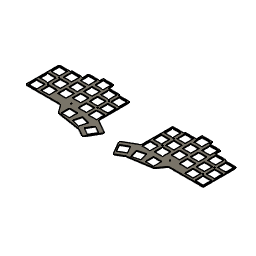
PlateV3 (Autodesk Fusion 360 design; units mm, degrees)
Autodesk Fusion 360 part; units mm, degrees
(part 1 of 4)
sketch "v1" plane through (0, 0, 0) normal (0, 1, 0) x (1, 0, 0)
  line L0 (60.175, -2.525) -> (73.175, -2.525)
  line L1 (60.175, -16.525) -> (73.175, -16.525)
  line L2 (59.675, -3.025) -> (59.675, -16.025)
  line L3 (73.675, -3.025) -> (73.675, -16.025)
  arc A0 (60.175, -2.525) -> (59.675, -3.025) centre (60.175, -3.025) ccw
  arc A1 (73.675, -3.025) -> (73.175, -2.525) centre (73.175, -3.025) ccw
  arc A2 (59.675, -16.025) -> (60.175, -16.525) centre (60.175, -16.025) ccw
  arc A3 (73.175, -16.525) -> (73.675, -16.025) centre (73.175, -16.025) ccw
  line L4 (41.125, -10.145) -> (54.125, -10.145)
  line L5 (41.125, -24.145) -> (54.125, -24.145)
  line L6 (40.625, -10.645) -> (40.625, -23.645)
  line L7 (54.625, -10.645) -> (54.625, -23.645)
  arc A4 (41.125, -10.145) -> (40.625, -10.645) centre (41.125, -10.645) ccw
  arc A5 (54.625, -10.645) -> (54.125, -10.145) centre (54.125, -10.645) ccw
  arc A6 (40.625, -23.645) -> (41.125, -24.145) centre (41.125, -23.645) ccw
  arc A7 (54.125, -24.145) -> (54.625, -23.645) centre (54.125, -23.645) ccw
  line L8 (79.225, -13.955) -> (92.225, -13.955)
  line L9 (79.225, -27.955) -> (92.225, -27.955)
  line L10 (78.725, -14.455) -> (78.725, -27.455)
  line L11 (92.725, -14.455) -> (92.725, -27.455)
  arc A8 (79.225, -13.955) -> (78.725, -14.455) centre (79.225, -14.455) ccw
  arc A9 (92.725, -14.455) -> (92.225, -13.955) centre (92.225, -14.455) ccw
  arc A10 (78.725, -27.455) -> (79.225, -27.955) centre (79.225, -27.455) ccw
  arc A11 (92.225, -27.955) -> (92.725, -27.455) centre (92.225, -27.455) ccw
  line L12 (98.275, -15.86) -> (111.275, -15.86)
  line L13 (98.275, -29.86) -> (111.275, -29.86)
  line L14 (97.775, -16.36) -> (97.775, -29.36)
  line L15 (111.775, -16.36) -> (111.775, -29.36)
  arc A12 (98.275, -15.86) -> (97.775, -16.36) centre (98.275, -16.36) ccw
  arc A13 (111.775, -16.36) -> (111.275, -15.86) centre (111.275, -16.36) ccw
  arc A14 (97.775, -29.36) -> (98.275, -29.86) centre (98.275, -29.36) ccw
  arc A15 (111.275, -29.86) -> (111.775, -29.36) centre (111.275, -29.36) ccw
  line L16 (3.025, -16.8125) -> (16.025, -16.8125)
  line L17 (3.025, -30.8125) -> (16.025, -30.8125)
  line L18 (2.525, -17.3125) -> (2.525, -30.3125)
  line L19 (16.525, -17.3125) -> (16.525, -30.3125)
  arc A16 (3.025, -16.8125) -> (2.525, -17.3125) centre (3.025, -17.3125) ccw
  arc A17 (16.525, -17.3125) -> (16.025, -16.8125) centre (16.025, -17.3125) ccw
  arc A18 (2.525, -30.3125) -> (3.025, -30.8125) centre (3.025, -30.3125) ccw
  arc A19 (16.025, -30.8125) -> (16.525, -30.3125) centre (16.025, -30.3125) ccw
  line L20 (22.075, -16.8125) -> (35.075, -16.8125)
  line L21 (22.075, -30.8125) -> (35.075, -30.8125)
  line L22 (21.575, -17.3125) -> (21.575, -30.3125)
  line L23 (35.575, -17.3125) -> (35.575, -30.3125)
  arc A20 (22.075, -16.8125) -> (21.575, -17.3125) centre (22.075, -17.3125) ccw
  arc A21 (35.575, -17.3125) -> (35.075, -16.8125) centre (35.075, -17.3125) ccw
  arc A22 (21.575, -30.3125) -> (22.075, -30.8125) centre (22.075, -30.3125) ccw
  arc A23 (35.075, -30.8125) -> (35.575, -30.3125) centre (35.075, -30.3125) ccw
  line L24 (60.175, -21.575) -> (73.175, -21.575)
  line L25 (60.175, -35.575) -> (73.175, -35.575)
  line L26 (59.675, -22.075) -> (59.675, -35.075)
  line L27 (73.675, -22.075) -> (73.675, -35.075)
  arc A24 (60.175, -21.575) -> (59.675, -22.075) centre (60.175, -22.075) ccw
  arc A25 (73.675, -22.075) -> (73.175, -21.575) centre (73.175, -22.075) ccw
  arc A26 (59.675, -35.075) -> (60.175, -35.575) centre (60.175, -35.075) ccw
  arc A27 (73.175, -35.575) -> (73.675, -35.075) centre (73.175, -35.075) ccw
  line L28 (41.125, -29.195) -> (54.125, -29.195)
  line L29 (41.125, -43.195) -> (54.125, -43.195)
  line L30 (40.625, -29.695) -> (40.625, -42.695)
  line L31 (54.625, -29.695) -> (54.625, -42.695)
  arc A28 (41.125, -29.195) -> (40.625, -29.695) centre (41.125, -29.695) ccw
  arc A29 (54.625, -29.695) -> (54.125, -29.195) centre (54.125, -29.695) ccw
  arc A30 (40.625, -42.695) -> (41.125, -43.195) centre (41.125, -42.695) ccw
  arc A31 (54.125, -43.195) -> (54.625, -42.695) centre (54.125, -42.695) ccw
  line L32 (79.225, -33.005) -> (92.225, -33.005)
  line L33 (79.225, -47.005) -> (92.225, -47.005)
  line L34 (78.725, -33.505) -> (78.725, -46.505)
  line L35 (92.725, -33.505) -> (92.725, -46.505)
  arc A32 (79.225, -33.005) -> (78.725, -33.505) centre (79.225, -33.505) ccw
  arc A33 (92.725, -33.505) -> (92.225, -33.005) centre (92.225, -33.505) ccw
  arc A34 (78.725, -46.505) -> (79.225, -47.005) centre (79.225, -46.505) ccw
  arc A35 (92.225, -47.005) -> (92.725, -46.505) centre (92.225, -46.505) ccw
  line L36 (98.275, -34.91) -> (111.275, -34.91)
  line L37 (98.275, -48.91) -> (111.275, -48.91)
  line L38 (97.775, -35.41) -> (97.775, -48.41)
  line L39 (111.775, -35.41) -> (111.775, -48.41)
  arc A36 (98.275, -34.91) -> (97.775, -35.41) centre (98.275, -35.41) ccw
  arc A37 (111.775, -35.41) -> (111.275, -34.91) centre (111.275, -35.41) ccw
  arc A38 (97.775, -48.41) -> (98.275, -48.91) centre (98.275, -48.41) ccw
  arc A39 (111.275, -48.91) -> (111.775, -48.41) centre (111.275, -48.41) ccw
  line L40 (3.025, -35.8625) -> (16.025, -35.8625)
  line L41 (3.025, -49.8625) -> (16.025, -49.8625)
  line L42 (2.525, -36.3625) -> (2.525, -49.3625)
  line L43 (16.525, -36.3625) -> (16.525, -49.3625)
  arc A40 (3.025, -35.8625) -> (2.525, -36.3625) centre (3.025, -36.3625) ccw
  arc A41 (16.525, -36.3625) -> (16.025, -35.8625) centre (16.025, -36.3625) ccw
  arc A42 (2.525, -49.3625) -> (3.025, -49.8625) centre (3.025, -49.3625) ccw
  arc A43 (16.025, -49.8625) -> (16.525, -49.3625) centre (16.025, -49.3625) ccw
  line L44 (22.075, -35.8625) -> (35.075, -35.8625)
  line L45 (22.075, -49.8625) -> (35.075, -49.8625)
  line L46 (21.575, -36.3625) -> (21.575, -49.3625)
  line L47 (35.575, -36.3625) -> (35.575, -49.3625)
  arc A44 (22.075, -35.8625) -> (21.575, -36.3625) centre (22.075, -36.3625) ccw
  arc A45 (35.575, -36.3625) -> (35.075, -35.8625) centre (35.075, -36.3625) ccw
  arc A46 (21.575, -49.3625) -> (22.075, -49.8625) centre (22.075, -49.3625) ccw
  arc A47 (35.075, -49.8625) -> (35.575, -49.3625) centre (35.075, -49.3625) ccw
  line L48 (60.175, -40.625) -> (73.175, -40.625)
  line L49 (60.175, -54.625) -> (73.175, -54.625)
  line L50 (59.675, -41.125) -> (59.675, -54.125)
  line L51 (73.675, -41.125) -> (73.675, -54.125)
  arc A48 (60.175, -40.625) -> (59.675, -41.125) centre (60.175, -41.125) ccw
  arc A49 (73.675, -41.125) -> (73.175, -40.625) centre (73.175, -41.125) ccw
  arc A50 (59.675, -54.125) -> (60.175, -54.625) centre (60.175, -54.125) ccw
  arc A51 (73.175, -54.625) -> (73.675, -54.125) centre (73.175, -54.125) ccw
  line L52 (41.125, -48.245) -> (54.125, -48.245)
  line L53 (41.125, -62.245) -> (54.125, -62.245)
  line L54 (40.625, -48.745) -> (40.625, -61.745)
  line L55 (54.625, -48.745) -> (54.625, -61.745)
  arc A52 (41.125, -48.245) -> (40.625, -48.745) centre (41.125, -48.745) ccw
  arc A53 (54.625, -48.745) -> (54.125, -48.245) centre (54.125, -48.745) ccw
  arc A54 (40.625, -61.745) -> (41.125, -62.245) centre (41.125, -61.745) ccw
  arc A55 (54.125, -62.245) -> (54.625, -61.745) centre (54.125, -61.745) ccw
  line L56 (79.225, -52.055) -> (92.225, -52.055)
  line L57 (79.225, -66.055) -> (92.225, -66.055)
  line L58 (78.725, -52.555) -> (78.725, -65.555)
  line L59 (92.725, -52.555) -> (92.725, -65.555)
  arc A56 (79.225, -52.055) -> (78.725, -52.555) centre (79.225, -52.555) ccw
  arc A57 (92.725, -52.555) -> (92.225, -52.055) centre (92.225, -52.555) ccw
  arc A58 (78.725, -65.555) -> (79.225, -66.055) centre (79.225, -65.555) ccw
  arc A59 (92.225, -66.055) -> (92.725, -65.555) centre (92.225, -65.555) ccw
  line L60 (98.275, -53.96) -> (111.275, -53.96)
  line L61 (98.275, -67.96) -> (111.275, -67.96)
  line L62 (97.775, -54.46) -> (97.775, -67.46)
  line L63 (111.775, -54.46) -> (111.775, -67.46)
  arc A60 (98.275, -53.96) -> (97.775, -54.46) centre (98.275, -54.46) ccw
  arc A61 (111.775, -54.46) -> (111.275, -53.96) centre (111.275, -54.46) ccw
  arc A62 (97.775, -67.46) -> (98.275, -67.96) centre (98.275, -67.46) ccw
  arc A63 (111.275, -67.96) -> (111.775, -67.46) centre (111.275, -67.46) ccw
  line L64 (3.025, -54.9125) -> (16.025, -54.9125)
  line L65 (3.025, -68.9125) -> (16.025, -68.9125)
  line L66 (2.525, -55.4125) -> (2.525, -68.4125)
  line L67 (16.525, -55.4125) -> (16.525, -68.4125)
  arc A64 (3.025, -54.9125) -> (2.525, -55.4125) centre (3.025, -55.4125) ccw
  arc A65 (16.525, -55.4125) -> (16.025, -54.9125) centre (16.025, -55.4125) ccw
  arc A66 (2.525, -68.4125) -> (3.025, -68.9125) centre (3.025, -68.4125) ccw
  arc A67 (16.025, -68.9125) -> (16.525, -68.4125) centre (16.025, -68.4125) ccw
  line L68 (22.075, -54.9125) -> (35.075, -54.9125)
  line L69 (22.075, -68.9125) -> (35.075, -68.9125)
  line L70 (21.575, -55.4125) -> (21.575, -68.4125)
  line L71 (35.575, -55.4125) -> (35.575, -68.4125)
  arc A68 (22.075, -54.9125) -> (21.575, -55.4125) centre (22.075, -55.4125) ccw
  arc A69 (35.575, -55.4125) -> (35.075, -54.9125) centre (35.075, -55.4125) ccw
  arc A70 (21.575, -68.4125) -> (22.075, -68.9125) centre (22.075, -68.4125) ccw
  arc A71 (35.075, -68.9125) -> (35.575, -68.4125) centre (35.075, -68.4125) ccw
  line L72 (69.7, -73.9625) -> (82.7, -73.9625)
  line L73 (69.7, -87.9625) -> (82.7, -87.9625)
  line L74 (69.2, -74.4625) -> (69.2, -87.4625)
  line L75 (83.2, -74.4625) -> (83.2, -87.4625)
  arc A72 (69.7, -73.9625) -> (69.2, -74.4625) centre (69.7, -74.4625) ccw
  arc A73 (83.2, -74.4625) -> (82.7, -73.9625) centre (82.7, -74.4625) ccw
  arc A74 (69.2, -87.4625) -> (69.7, -87.9625) centre (69.7, -87.4625) ccw
  arc A75 (82.7, -87.9625) -> (83.2, -87.4625) centre (82.7, -87.4625) ccw
  line L76 (94.5706, -75.2238) -> (107.1276, -78.5884)
  line L77 (90.9471, -88.7468) -> (103.5041, -92.1114)
  line L78 (93.9582, -75.5774) -> (90.5936, -88.1344)
  line L79 (107.4812, -79.2008) -> (104.1165, -91.7579)
  arc A76 (94.5706, -75.2238) -> (93.9582, -75.5774) centre (94.4412, -75.7068) ccw
  arc A77 (107.4812, -79.2008) -> (107.1276, -78.5884) centre (106.9982, -79.0714) ccw
  arc A78 (90.5936, -88.1344) -> (90.9471, -88.7468) centre (91.0765, -88.2638) ccw
  arc A79 (103.5041, -92.1114) -> (104.1165, -91.7579) centre (103.6336, -91.6284) ccw
  line L80 (132.3373, -85.6651) -> (125.8373, -96.9234)
  line L81 (120.213, -78.6651) -> (113.713, -89.9234)
  line L82 (132.1543, -84.9821) -> (120.896, -78.4821)
  line L83 (125.1543, -97.1064) -> (113.896, -90.6064)
  arc A80 (132.3373, -85.6651) -> (132.1543, -84.9821) centre (131.9043, -85.4151) ccw
  arc A81 (125.1543, -97.1064) -> (125.8373, -96.9234) centre (125.4043, -96.6734) ccw
  arc A82 (120.896, -78.4821) -> (120.213, -78.6651) centre (120.646, -78.9151) ccw
  arc A83 (113.713, -89.9234) -> (113.896, -90.6064) centre (114.146, -90.1734) ccw
  line L84 (1.025, -14.8125) -> (16.025, -14.8125)
  line L85 (22.075, -14.8125) -> (38.125, -14.8125)
  line L86 (41.125, -8.145) -> (57.175, -8.145)
  line L87 (58.175, -0.525) -> (73.175, -0.525)
  line L88 (76.175, -11.955) -> (92.225, -11.955)
  line L89 (95.225, -13.86) -> (113.275, -13.86)
  line L90 (113.775, -35.41) -> (113.775, -48.41)
  line L91 (113.775, -14.36) -> (113.775, -29.36)
  line L92 (113.775, -54.46) -> (113.775, -70.3293)
  line L93 (134.8864, -84.25) -> (115.275, -72.9274)
  line L94 (135.0694, -84.933) -> (126.4078, -99.9353)
  line L95 (88.3927, -90.1329) -> (102.9865, -94.0433)
  line L96 (70.2949, -89.9625) -> (87.0986, -89.9625)
  line L97 (22.075, -70.9125) -> (35.1033, -70.9125)
  line L98 (1.025, -70.9125) -> (16.025, -70.9125)
  line L99 (0.525, -55.4125) -> (0.525, -70.4125)
  line L100 (0.525, -36.3625) -> (0.525, -49.3625)
  line L101 (0.525, -15.3125) -> (0.525, -30.3125)
  line L102 (0.525, -30.3125) -> (0.525, -36.3625)
  line L103 (0.525, -49.3625) -> (0.525, -55.4125)
  line L104 (16.025, -70.9125) -> (22.075, -70.9125)
  line L105 (113.775, -54.46) -> (113.775, -48.41)
  line L106 (113.775, -35.41) -> (113.775, -29.36)
  line L107 (16.025, -14.8125) -> (22.075, -14.8125)
  line L108 (70.5671, -89.9625) -> (68.5671, -89.9625)
  line L109 (35.1033, -70.9125) -> (37.1033, -70.9125)
  line L110 (37.1033, -70.9125) -> (54.6027, -70.8754)
  line L111 (58.9382, -73.3662) -> (67.7, -88.468)
  line L112 (102.9865, -94.0433) -> (125.8454, -100.1683)
  line L113 (126.216, -100.2676) -> (127.5694, -97.9234)
  arc A84 (88.3927, -90.1329) -> (87.0986, -89.9625) centre (87.0986, -94.9625) ccw
  arc A85 (135.0694, -84.933) -> (134.8864, -84.25) centre (134.6364, -84.683) ccw
  arc A86 (113.775, -70.3293) -> (115.275, -72.9274) centre (116.775, -70.3293) ccw
  arc A87 (113.775, -14.36) -> (113.275, -13.86) centre (113.275, -14.36) ccw
  arc A88 (58.9382, -73.3662) -> (54.6027, -70.8754) centre (54.6133, -75.8753) ccw
  arc A89 (67.7, -88.468) -> (70.2949, -89.9625) centre (70.2949, -86.9625) ccw
  arc A90 (0.525, -70.4125) -> (1.025, -70.9125) centre (1.025, -70.4125) ccw
  arc A91 (1.025, -14.8125) -> (0.525, -15.3125) centre (1.025, -15.3125) ccw
  arc A92 (125.8454, -100.1683) -> (126.4078, -99.9353) centre (125.9748, -99.6853) ccw
  line L114 (38.625, -14.3125) -> (38.625, -8.645)
  line L115 (41.125, -8.145) -> (39.125, -8.145)
  line L116 (57.675, -7.645) -> (57.675, -1.025)
  line L117 (57.675, -0.525) -> (60.175, -0.525)
  line L118 (75.675, -11.455) -> (75.675, -1.025)
  line L119 (75.175, -0.525) -> (73.175, -0.525)
  line L120 (94.725, -13.36) -> (94.725, -12.455)
  line L121 (94.225, -11.955) -> (92.225, -11.955)
  arc A93 (38.125, -14.8125) -> (38.625, -14.3125) centre (38.125, -14.3125) ccw
  arc A94 (39.125, -8.145) -> (38.625, -8.645) centre (39.125, -8.645) ccw
  arc A95 (57.175, -8.145) -> (57.675, -7.645) centre (57.175, -7.645) ccw
  arc A96 (58.175, -0.525) -> (57.675, -1.025) centre (58.175, -1.025) ccw
  arc A97 (75.675, -1.025) -> (75.175, -0.525) centre (75.175, -1.025) ccw
  arc A98 (94.725, -12.455) -> (94.225, -11.955) centre (94.225, -12.455) ccw
  arc A99 (75.675, -11.455) -> (76.175, -11.955) centre (76.175, -11.455) ccw
  arc A100 (94.725, -13.36) -> (95.225, -13.86) centre (95.225, -13.36) ccw
  arc A101 (169.0598, -78.6651) -> (168.3767, -78.4821) centre (168.6267, -78.9151) ccw
  arc A102 (157.1184, -84.9821) -> (156.9354, -85.6651) centre (157.3684, -85.4151) ccw
  line L122 (181.7916, -79.2008) -> (185.1562, -91.7579)
  line L123 (154.3864, -84.25) -> (173.9977, -72.9274)
  line L124 (156.9354, -85.6651) -> (163.4354, -96.9234)
  arc A103 (162.8649, -99.9353) -> (163.4273, -100.1683) centre (163.2979, -99.6853) ccw
  arc A104 (190.9977, -67.96) -> (191.4977, -67.46) centre (190.9977, -67.46) ccw
  line L125 (230.3346, -73.3662) -> (221.5727, -88.468)
  line L126 (163.0567, -100.2676) -> (161.7033, -97.9234)
  line L127 (154.2033, -84.933) -> (162.8649, -99.9353)
  line L128 (229.0977, -2.525) -> (216.0977, -2.525)
  arc A105 (177.9977, -53.96) -> (177.4977, -54.46) centre (177.9977, -54.46) ccw
  line L129 (157.1184, -84.9821) -> (168.3767, -78.4821)
  line L130 (229.0977, -16.525) -> (216.0977, -16.525)
  line L131 (190.9977, -67.96) -> (177.9977, -67.96)
  line L132 (229.0977, -54.625) -> (216.0977, -54.625)
  line L133 (196.5477, -33.505) -> (196.5477, -46.505)
  line L134 (190.9977, -48.91) -> (177.9977, -48.91)
  line L135 (229.0977, -21.575) -> (216.0977, -21.575)
  line L136 (229.0977, -40.625) -> (216.0977, -40.625)
  line L137 (253.6977, -36.3625) -> (253.6977, -49.3625)
  line L138 (229.5977, -41.125) -> (229.5977, -54.125)
  line L139 (267.6977, -36.3625) -> (267.6977, -49.3625)
  line L140 (215.5977, -41.125) -> (215.5977, -54.125)
  line L141 (210.5477, -33.505) -> (210.5477, -46.505)
  line L142 (288.7477, -36.3625) -> (288.7477, -49.3625)
  line L143 (177.4977, -35.41) -> (177.4977, -48.41)
  line L144 (175.4977, -35.41) -> (175.4977, -48.41)
  line L145 (286.7477, -36.3625) -> (286.7477, -49.3625)
  line L146 (194.7021, -75.2238) -> (182.1451, -78.5884)
  line L147 (272.7477, -36.3625) -> (272.7477, -49.3625)
  line L148 (191.4977, -35.41) -> (191.4977, -48.41)
  line L149 (164.1184, -97.1064) -> (175.3767, -90.6064)
  line L150 (190.9977, -53.96) -> (177.9977, -53.96)
  arc A106 (177.4977, -48.41) -> (177.9977, -48.91) centre (177.9977, -48.41) ccw
  line L151 (248.1477, -29.195) -> (235.1477, -29.195)
  arc A107 (267.1977, -68.9125) -> (267.6977, -68.4125) centre (267.1977, -68.4125) ccw
  line L152 (288.7477, -49.3625) -> (288.7477, -55.4125)
  arc A108 (272.7477, -68.4125) -> (273.2477, -68.9125) centre (273.2477, -68.4125) ccw
  arc A109 (196.5477, -27.455) -> (197.0477, -27.955) centre (197.0477, -27.455) ccw
  line L153 (288.7477, -15.3125) -> (288.7477, -30.3125)
  line L154 (210.0477, -33.005) -> (197.0477, -33.005)
  line L155 (286.2477, -16.8125) -> (273.2477, -16.8125)
  arc A110 (248.6477, -10.645) -> (248.1477, -10.145) centre (248.1477, -10.645) ccw
  arc A111 (213.0977, -11.955) -> (213.5977, -11.455) centre (213.0977, -11.455) ccw
  arc A112 (215.5977, -35.075) -> (216.0977, -35.575) centre (216.0977, -35.075) ccw
  arc A113 (210.0477, -47.005) -> (210.5477, -46.505) centre (210.0477, -46.505) ccw
  line L156 (288.2477, -70.9125) -> (273.2477, -70.9125)
  line L157 (272.7477, -17.3125) -> (272.7477, -30.3125)
  arc A114 (267.1977, -30.8125) -> (267.6977, -30.3125) centre (267.1977, -30.3125) ccw
  line L158 (286.7477, -17.3125) -> (286.7477, -30.3125)
  arc A115 (197.0477, -52.055) -> (196.5477, -52.555) centre (197.0477, -52.555) ccw
  line L159 (213.0977, -11.955) -> (197.0477, -11.955)
  arc A116 (267.6977, -17.3125) -> (267.1977, -16.8125) centre (267.1977, -17.3125) ccw
  arc A117 (272.7477, -30.3125) -> (273.2477, -30.8125) centre (273.2477, -30.3125) ccw
  line L160 (229.5977, -3.025) -> (229.5977, -16.025)
  arc A118 (273.2477, -16.8125) -> (272.7477, -17.3125) centre (273.2477, -17.3125) ccw
  arc A119 (273.2477, -54.9125) -> (272.7477, -55.4125) centre (273.2477, -55.4125) ccw
  line L161 (215.5977, -3.025) -> (215.5977, -16.025)
  line L162 (210.0477, -27.955) -> (197.0477, -27.955)
  arc A120 (216.0977, -40.625) -> (215.5977, -41.125) centre (216.0977, -41.125) ccw
  arc A121 (235.1477, -10.145) -> (234.6477, -10.645) centre (235.1477, -10.645) ccw
  arc A122 (210.0477, -27.955) -> (210.5477, -27.455) centre (210.0477, -27.455) ccw
  line L163 (288.7477, -30.3125) -> (288.7477, -36.3625)
  arc A123 (286.2477, -30.8125) -> (286.7477, -30.3125) centre (286.2477, -30.3125) ccw
  line L164 (273.2477, -14.8125) -> (267.1977, -14.8125)
  arc A124 (254.1977, -16.8125) -> (253.6977, -17.3125) centre (254.1977, -17.3125) ccw
  line L165 (229.5977, -22.075) -> (229.5977, -35.075)
  arc A125 (253.6977, -30.3125) -> (254.1977, -30.8125) centre (254.1977, -30.3125) ccw
  arc A126 (286.7477, -17.3125) -> (286.2477, -16.8125) centre (286.2477, -17.3125) ccw
  arc A127 (254.1977, -35.8625) -> (253.6977, -36.3625) centre (254.1977, -36.3625) ccw
  line L166 (288.2477, -14.8125) -> (273.2477, -14.8125)
  arc A128 (248.6477, -29.695) -> (248.1477, -29.195) centre (248.1477, -29.695) ccw
  arc A129 (250.6477, -14.3125) -> (251.1477, -14.8125) centre (251.1477, -14.3125) ccw
  line L167 (234.6477, -10.645) -> (234.6477, -23.645)
  arc A130 (231.5977, -7.645) -> (232.0977, -8.145) centre (232.0977, -7.645) ccw
  arc A131 (288.7477, -15.3125) -> (288.2477, -14.8125) centre (288.2477, -15.3125) ccw
  line L168 (267.6977, -17.3125) -> (267.6977, -30.3125)
  arc A132 (210.5477, -33.505) -> (210.0477, -33.005) centre (210.0477, -33.505) ccw
  line L169 (248.1477, -8.145) -> (232.0977, -8.145)
  line L170 (286.2477, -35.8625) -> (273.2477, -35.8625)
  arc A133 (229.5977, -22.075) -> (229.0977, -21.575) centre (229.0977, -22.075) ccw
  line L171 (253.6977, -17.3125) -> (253.6977, -30.3125)
  line L172 (248.6477, -10.645) -> (248.6477, -23.645)
  line L173 (248.1477, -8.145) -> (250.1477, -8.145)
  arc A134 (248.1477, -43.195) -> (248.6477, -42.695) centre (248.1477, -42.695) ccw
  line L174 (231.5977, -7.645) -> (231.5977, -1.025)
  arc A135 (248.1477, -24.145) -> (248.6477, -23.645) centre (248.1477, -23.645) ccw
  line L175 (231.5977, -0.525) -> (229.0977, -0.525)
  arc A136 (234.6477, -42.695) -> (235.1477, -43.195) centre (235.1477, -42.695) ccw
  arc A137 (235.1477, -29.195) -> (234.6477, -29.695) centre (235.1477, -29.695) ccw
  line L176 (234.6477, -29.695) -> (234.6477, -42.695)
  arc A138 (229.5977, -41.125) -> (229.0977, -40.625) centre (229.0977, -41.125) ccw
  line L177 (250.6477, -14.3125) -> (250.6477, -8.645)
  arc A139 (229.0977, -16.525) -> (229.5977, -16.025) centre (229.0977, -16.025) ccw
  line L178 (248.1477, -10.145) -> (235.1477, -10.145)
  arc A140 (229.0977, -35.575) -> (229.5977, -35.075) centre (229.0977, -35.075) ccw
  arc A141 (231.5977, -1.025) -> (231.0977, -0.525) centre (231.0977, -1.025) ccw
  line L179 (248.6477, -29.695) -> (248.6477, -42.695)
  arc A142 (173.9977, -72.9274) -> (175.4977, -70.3293) centre (172.4977, -70.3293) ccw
  line L180 (175.4977, -54.46) -> (175.4977, -48.41)
  arc A143 (185.1562, -91.7579) -> (185.7686, -92.1114) centre (185.6392, -91.6284) ccw
  arc A144 (191.4977, -54.46) -> (190.9977, -53.96) centre (190.9977, -54.46) ccw
  line L181 (169.0598, -78.6651) -> (175.5598, -89.9234)
  arc A145 (154.3864, -84.25) -> (154.2033, -84.933) centre (154.6364, -84.683) ccw
  line L182 (177.4977, -54.46) -> (177.4977, -67.46)
  line L183 (190.9977, -29.86) -> (177.9977, -29.86)
  line L184 (267.1977, -68.9125) -> (254.1977, -68.9125)
  line L185 (267.1977, -54.9125) -> (254.1977, -54.9125)
  line L186 (267.1977, -30.8125) -> (254.1977, -30.8125)
  line L187 (267.1977, -49.8625) -> (254.1977, -49.8625)
  line L188 (210.0477, -47.005) -> (197.0477, -47.005)
  line L189 (195.0477, -11.955) -> (197.0477, -11.955)
  line L190 (248.6477, -48.745) -> (248.6477, -61.745)
  arc A146 (196.5477, -65.555) -> (197.0477, -66.055) centre (197.0477, -65.555) ccw
  line L191 (218.7056, -89.9625) -> (220.7056, -89.9625)
  arc A147 (195.3145, -75.5774) -> (194.7021, -75.2238) centre (194.8316, -75.7068) ccw
  line L192 (267.1977, -16.8125) -> (254.1977, -16.8125)
  arc A148 (215.5977, -54.125) -> (216.0977, -54.625) centre (216.0977, -54.125) ccw
  arc A149 (253.6977, -49.3625) -> (254.1977, -49.8625) centre (254.1977, -49.3625) ccw
  line L193 (215.5977, -22.075) -> (215.5977, -35.075)
  line L194 (200.88, -90.1329) -> (186.2862, -94.0433)
  arc A150 (195.0477, -11.955) -> (194.5477, -12.455) centre (195.0477, -12.455) ccw
  line L195 (196.5477, -14.455) -> (196.5477, -27.455)
  arc A151 (177.9977, -15.86) -> (177.4977, -16.36) centre (177.9977, -16.36) ccw
  line L196 (198.3256, -88.7468) -> (185.7686, -92.1114)
  line L197 (194.0477, -13.86) -> (175.9977, -13.86)
  arc A152 (229.0977, -54.625) -> (229.5977, -54.125) centre (229.0977, -54.125) ccw
  line L198 (267.1977, -70.9125) -> (254.1694, -70.9125)
  line L199 (195.3145, -75.5774) -> (198.6792, -88.1344)
  line L200 (286.2477, -68.9125) -> (273.2477, -68.9125)
  line L201 (219.5727, -73.9625) -> (206.5727, -73.9625)
  line L202 (248.1477, -62.245) -> (235.1477, -62.245)
  arc A153 (197.0477, -33.005) -> (196.5477, -33.505) centre (197.0477, -33.505) ccw
  arc A154 (267.1977, -49.8625) -> (267.6977, -49.3625) centre (267.1977, -49.3625) ccw
  arc A155 (234.6477, -61.745) -> (235.1477, -62.245) centre (235.1477, -61.745) ccw
  arc A156 (198.3256, -88.7468) -> (198.6792, -88.1344) centre (198.1962, -88.2638) ccw
  arc A157 (191.4977, -16.36) -> (190.9977, -15.86) centre (190.9977, -16.36) ccw
  arc A158 (286.2477, -68.9125) -> (286.7477, -68.4125) centre (286.2477, -68.4125) ccw
  line L203 (175.4977, -14.36) -> (175.4977, -29.36)
  line L204 (194.5477, -13.36) -> (194.5477, -12.455)
  line L205 (267.1977, -14.8125) -> (251.1477, -14.8125)
  line L206 (234.6477, -48.745) -> (234.6477, -61.745)
  arc A159 (194.0477, -13.86) -> (194.5477, -13.36) centre (194.0477, -13.36) ccw
  line L207 (267.1977, -35.8625) -> (254.1977, -35.8625)
  line L208 (286.2477, -30.8125) -> (273.2477, -30.8125)
  arc A160 (177.9977, -34.91) -> (177.4977, -35.41) centre (177.9977, -35.41) ccw
  arc A161 (248.1477, -62.245) -> (248.6477, -61.745) centre (248.1477, -61.745) ccw
  line L209 (210.5477, -52.555) -> (210.5477, -65.555)
  arc A162 (248.6477, -48.745) -> (248.1477, -48.245) centre (248.1477, -48.745) ccw
  arc A163 (196.5477, -46.505) -> (197.0477, -47.005) centre (197.0477, -46.505) ccw
  line L210 (219.5727, -87.9625) -> (206.5727, -87.9625)
  arc A164 (190.9977, -29.86) -> (191.4977, -29.36) centre (190.9977, -29.36) ccw
  arc A165 (220.0727, -74.4625) -> (219.5727, -73.9625) centre (219.5727, -74.4625) ccw
  line L211 (175.4977, -35.41) -> (175.4977, -29.36)
  arc A166 (254.1977, -54.9125) -> (253.6977, -55.4125) centre (254.1977, -55.4125) ccw
  line L212 (253.6977, -55.4125) -> (253.6977, -68.4125)
  arc A167 (216.0977, -21.575) -> (215.5977, -22.075) centre (216.0977, -22.075) ccw
  line L213 (288.7477, -55.4125) -> (288.7477, -70.4125)
  line L214 (252.1694, -70.9125) -> (234.67, -70.8754)
  arc A168 (218.9778, -89.9625) -> (221.5727, -88.468) centre (218.9778, -86.9625) ccw
  line L215 (248.1477, -48.245) -> (235.1477, -48.245)
  line L216 (196.5477, -52.555) -> (196.5477, -65.555)
  line L217 (272.7477, -55.4125) -> (272.7477, -68.4125)
  arc A169 (253.6977, -68.4125) -> (254.1977, -68.9125) centre (254.1977, -68.4125) ccw
  arc A170 (234.67, -70.8754) -> (230.3346, -73.3662) centre (234.6594, -75.8753) ccw
  line L218 (286.7477, -55.4125) -> (286.7477, -68.4125)
  arc A171 (210.0477, -66.055) -> (210.5477, -65.555) centre (210.0477, -65.555) ccw
  arc A172 (216.0977, -2.525) -> (215.5977, -3.025) centre (216.0977, -3.025) ccw
  arc A173 (191.4977, -35.41) -> (190.9977, -34.91) centre (190.9977, -35.41) ccw
  arc A174 (286.7477, -55.4125) -> (286.2477, -54.9125) centre (286.2477, -55.4125) ccw
  line L219 (190.9977, -34.91) -> (177.9977, -34.91)
  line L220 (254.1694, -70.9125) -> (252.1694, -70.9125)
  line L221 (286.2477, -49.8625) -> (273.2477, -49.8625)
  arc A175 (175.9977, -13.86) -> (175.4977, -14.36) centre (175.9977, -14.36) ccw
  arc A176 (177.4977, -29.36) -> (177.9977, -29.86) centre (177.9977, -29.36) ccw
  line L222 (218.9778, -89.9625) -> (202.1741, -89.9625)
  line L223 (220.0727, -74.4625) -> (220.0727, -87.4625)
  line L224 (210.0477, -13.955) -> (197.0477, -13.955)
  arc A177 (219.5727, -87.9625) -> (220.0727, -87.4625) centre (219.5727, -87.4625) ccw
  arc A178 (286.7477, -36.3625) -> (286.2477, -35.8625) centre (286.2477, -36.3625) ccw
  line L225 (214.0977, -0.525) -> (216.0977, -0.525)
  line L226 (248.1477, -43.195) -> (235.1477, -43.195)
  arc A179 (214.0977, -0.525) -> (213.5977, -1.025) centre (214.0977, -1.025) ccw
  arc A180 (229.5977, -3.025) -> (229.0977, -2.525) centre (229.0977, -3.025) ccw
  arc A181 (288.2477, -70.9125) -> (288.7477, -70.4125) centre (288.2477, -70.4125) ccw
  line L227 (248.1477, -24.145) -> (235.1477, -24.145)
  line L228 (213.5977, -11.455) -> (213.5977, -1.025)
  line L229 (190.9977, -15.86) -> (177.9977, -15.86)
  arc A182 (210.5477, -52.555) -> (210.0477, -52.055) centre (210.0477, -52.555) ccw
  line L230 (206.0727, -74.4625) -> (206.0727, -87.4625)
  arc A183 (235.1477, -48.245) -> (234.6477, -48.745) centre (235.1477, -48.745) ccw
  line L231 (210.0477, -52.055) -> (197.0477, -52.055)
  arc A184 (215.5977, -16.025) -> (216.0977, -16.525) centre (216.0977, -16.025) ccw
  line L232 (177.4977, -16.36) -> (177.4977, -29.36)
  arc A185 (197.0477, -13.955) -> (196.5477, -14.455) centre (197.0477, -14.455) ccw
  arc A186 (206.5727, -73.9625) -> (206.0727, -74.4625) centre (206.5727, -74.4625) ccw
  arc A187 (267.6977, -55.4125) -> (267.1977, -54.9125) centre (267.1977, -55.4125) ccw
  line L233 (191.4977, -16.36) -> (191.4977, -29.36)
  arc A188 (273.2477, -35.8625) -> (272.7477, -36.3625) centre (273.2477, -36.3625) ccw
  arc A189 (286.2477, -49.8625) -> (286.7477, -49.3625) centre (286.2477, -49.3625) ccw
  line L234 (273.2477, -70.9125) -> (267.1977, -70.9125)
  arc A190 (206.0727, -87.4625) -> (206.5727, -87.9625) centre (206.5727, -87.4625) ccw
  arc A191 (272.7477, -49.3625) -> (273.2477, -49.8625) centre (273.2477, -49.3625) ccw
  arc A192 (267.6977, -36.3625) -> (267.1977, -35.8625) centre (267.1977, -36.3625) ccw
  arc A193 (202.1741, -89.9625) -> (200.88, -90.1329) centre (202.1741, -94.9625) ccw
  line L235 (286.2477, -54.9125) -> (273.2477, -54.9125)
  line L236 (267.6977, -55.4125) -> (267.6977, -68.4125)
  line L237 (210.0477, -66.055) -> (197.0477, -66.055)
  arc A194 (250.6477, -8.645) -> (250.1477, -8.145) centre (250.1477, -8.645) ccw
  arc A195 (234.6477, -23.645) -> (235.1477, -24.145) centre (235.1477, -23.645) ccw
  arc A196 (210.5477, -14.455) -> (210.0477, -13.955) centre (210.0477, -14.455) ccw
  line L238 (210.5477, -14.455) -> (210.5477, -27.455)
  arc A197 (177.4977, -67.46) -> (177.9977, -67.96) centre (177.9977, -67.46) ccw
  line L239 (229.0977, -35.575) -> (216.0977, -35.575)
  arc A198 (163.4354, -96.9234) -> (164.1184, -97.1064) centre (163.8684, -96.6734) ccw
  arc A199 (190.9977, -48.91) -> (191.4977, -48.41) centre (190.9977, -48.41) ccw
  line L240 (231.0977, -0.525) -> (216.0977, -0.525)
  line L241 (186.2862, -94.0433) -> (163.4273, -100.1683)
  arc A200 (175.3767, -90.6064) -> (175.5598, -89.9234) centre (175.1267, -90.1734) ccw
  line L242 (175.4977, -54.46) -> (175.4977, -70.3293)
  line L243 (191.4977, -54.46) -> (191.4977, -67.46)
  arc A201 (182.1451, -78.5884) -> (181.7916, -79.2008) centre (182.2745, -79.0714) ccw
  point P0 (38.625, -14.8125)
  point P1 (57.675, -8.145)
  point P2 (75.675, -11.955)
  point P3 (94.725, -13.86)
  point P4 (213.5977, -11.955)
  point P5 (194.5477, -13.86)
  point P6 (231.5977, -8.145)
  point P7 (250.6477, -14.8125)
  dimension "d8" = -2
  dimension "d18" = 2
  dimension "d21" = 2
  dimension "d23" = 2
  dimension "d24" = 2
  dimension "d25" = 120
  dimension "d26" = 5
  dimension "d27" = 0.5
  dimension "d28" = 3
  dimension "d29" = 0.5
  dimension "d30" = 5
  dimension "d31" = 3
  dimension "d32" = 0.5
  dimension "d33" = 0.5
  dimension "d34" = 0.5
  dimension "d35" = 2
  dimension "d36" = 2
  dimension "d37" = 2
  dimension "d38" = 2
  dimension "d39" = 0.5
  dimension "d40" = 0.5
  dimension "d41" = 0.5
  dimension "d42" = 0.5
  dimension "d43" = 0.5
  dimension "d44" = 0.5
  dimension "d45" = 0.5
  dimension "d46" = 0.5
  dimension "d47" = 2
  constraint parallel L100 L102
  constraint perpendicular L41 L103
  constraint perpendicular L103 L104
  constraint perpendicular L104 L105
  constraint parallel L91 L106
  constraint perpendicular L106 L107
  constraint parallel L96 L108
  constraint parallel L97 L109
  constraint parallel L95 L112
  constraint parallel L94 L113
  constraint tangent L96 A84
  constraint tangent L95 A84
  constraint tangent L93 A85
  constraint tangent L94 A85
  constraint tangent L92 A86
  constraint tangent L93 A86
  constraint tangent L89 A87
  constraint tangent L91 A87
  constraint tangent L110 A88
  constraint tangent L111 A88
  constraint coincident L108.end L111
  constraint coincident L108.start L96
  constraint tangent L111 A89
  constraint tangent L96 A89
  constraint tangent L99 A90
  constraint tangent L98 A90
  constraint tangent L101 A91
  constraint tangent L84 A91
  constraint coincident L113.start L112
  constraint tangent L112 A92
  constraint tangent L94 A92
  constraint perpendicular L86 L114
  constraint perpendicular L114 L115
  constraint perpendicular L86 L116
  constraint perpendicular L7 L117
  constraint perpendicular L88 L118
  constraint perpendicular L118 L119
  constraint perpendicular L89 L120
  constraint perpendicular L120 L121
  constraint coincident P0 L85
  constraint coincident P0 L114
  constraint tangent L85 A93
  constraint tangent L114 A93
  constraint tangent L114 A94
  constraint tangent L115 A94
  constraint coincident P1 L86
  constraint coincident P1 L116
  constraint tangent L86 A95
  constraint tangent L116 A95
  constraint coincident L117.start L116
  constraint coincident L117.end L87
  constraint tangent L116 A96
  constraint tangent L87 A96
  constraint tangent L119 A97
  constraint tangent L118 A97
  constraint tangent L121 A98
  constraint tangent L120 A98
  constraint coincident P2 L118
  constraint coincident P2 L88
  constraint tangent L118 A99
  constraint tangent L88 A99
  constraint coincident P3 L120
  constraint coincident P3 L89
  constraint tangent L120 A100
  constraint tangent L89 A100
  measures "d23" distance of L108.start L108.end
  measures "d24" distance of L97.end L109.end
  measures "d25" angle of L110 L111
  measures "d26" radius of A84
  measures "d27" radius of A85
  measures "d28" radius of A86
  measures "d29" radius of A87
  measures "d30" radius of A88
  measures "d31" radius of A89
  measures "d32" radius of A90
  measures "d33" radius of A91
  measures "d34" radius of A92
  measures "d35" distance of L6 P0
  measures "d36" distance of L2 P1
  measures "d37" distance of L3 P2
  measures "d38" distance of L11 P3
  measures "d39" radius of A93
  measures "d40" radius of A94
  measures "d41" radius of A95
  measures "d42" radius of A96
  measures "d43" radius of A97
  measures "d44" radius of A98
  measures "d45" radius of A99
  measures "d46" radius of A100
  measures "d47" horizontal distance of L73.start L111.end
extrude "Extrude1" add sketch "v1" along normal blind 1.6 makes body 1 at (67.6, 0, 61.0932) makes body 2 at (221.6727, 0, 61.0932)